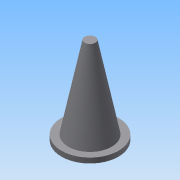
# Autodesk Inventor part: nozzlebottomcone
Saved by Autodesk Inventor 2015 SP1 (Build 190203100, 203)
## iProperties
Created: 2015-04-28
Part Number: nozzlebottomcone
Material: Generic
Document SubType Name: Modeling
Designer: Admin
Density: 1 g/cm^3
Appearance: Default
Author: Admin
Autodesk Inventor part; units mm, degrees
ref_plane "YZ Plane" through (0, 0, 0) normal (1, 0, 0) x (0, 1, 0)
ref_plane "XZ Plane" through (0, 0, 0) normal (0, 1, 0) x (-1, 0, 0)
ref_plane "XY Plane" through (0, 0, 0) normal (0, 0, 1) x (1, 0, 0)
sketch "Sketch1" plane through (0, 0, 0) normal (1, 0, 0) x (0, 1, 0)
  line L0 (0, 17.78) -> (3.175, 17.78)
  line L1 (3.175, 17.78) -> (3.175, 13.462)
  line L2 (0, 0) -> (54.229, 0)
  line L3 (0, 10.8337) -> (0, 17.78)
  line L4 (54.229, 0) -> (54.229, 3.302)
  line L5 (54.229, 3.302) -> (3.175, 13.462)
  line L6 (0, 10.8337) -> (51.4203, 0)
  dimension "d0" = 17.78
  dimension "d1" = 3.175
  dimension "d2" = 4.318
  dimension "d3" = 54.229
  dimension "d6" = 3.302
  constraints: 14 end point, 3 vertical, 2 horizontal, 1 point on line
  measures "d0" distance of L2.start L0.start
  measures "d1" distance of L0.start L0.end
  measures "d2" distance of L0.end L1.end
  measures "d3" distance of L2.start L2.end
  measures "d6" distance of L2.end L4.end
revolve "Revolution1" add sketch "Sketch1" angle 360 about axis through (0, 0, 0) along (0, 1, 0)
body "Solid1"
